Autodesk Fusion 360 part; units mm, degrees
(part 2 of 2)
sketch "Sketch1 (2)" plane through (5.45, -12.4, 0) normal (0, 1, 0) x (-1, 0, 0) in component "ServoTrayMount"
  line L0 (-16.2, -6.2) -> (-11.2, -6.2) construction
  line L1 (-16.2, 6.2) -> (-16.2, -6.2) construction
  line L2 (-16.2, -0.6) -> (-15.053256, -0.6) construction
  line L3 (-16.2, 0.6) -> (-15.053256, 0.6) construction
  circle A0 centre (-13.9, 0) radius 1.3
  line L4 (-11.2, 6.2) -> (-16.2, 6.2) construction
  line L5 (-11.2, 0) -> (-11.2, 12.4) construction
  line L6 (-11.2, 0) -> (-11.2, -12.4) construction
  line L7 (11.2, -6.2) -> (11.2, 0) construction
  line L8 (16.2, -6.2) -> (11.2, -6.2) construction
  line L9 (16.2, 6.2) -> (16.2, -6.2) construction
  line L10 (16.2, 0.6) -> (15.053256, 0.6) construction
  line L11 (16.2, -0.6) -> (15.053256, -0.6) construction
  circle A1 centre (13.9, 0) radius 1.3
  line L12 (11.2, 6.2) -> (11.2, 0) construction
  line L13 (11.2, 6.2) -> (16.2, 6.2) construction
  line L14 (-11.2, 6.2) -> (11.2, 6.2) construction
  line L15 (-11.2, -6.2) -> (11.2, -6.2) construction
  circle A2 centre (5.45, 0) radius 1.25
  line L16 (-16.2, -6.2) -> (-16.2, -6.4) construction
  line L17 (-16.2, -6.4) -> (-16.4, -6.4) construction
  line L18 (16.2, 6.2) -> (16.2, 6.4) construction
  line L19 (16.2, 6.4) -> (16.4, 6.4) construction
  line L20 (16.4, 6.4) -> (-16.4, 6.4)
  line L21 (-16.4, 6.4) -> (-16.4, -6.4)
  line L22 (-16.4, -6.4) -> (16.4, -6.4)
  line L23 (16.4, -6.4) -> (16.4, 6.4)
  line L24 (-16.4, -6.4) -> (-16.4, -9.4) construction
  line L25 (-11.2, -6.4) -> (-11.4, -6.4)
  line L26 (-11.4, -6.4) -> (-11.4, 6.4)
  line L27 (0, -6.2) -> (0, 6.2) construction
  line L28 (11.4, -6.4) -> (11.4, 6.4)
  line L29 (-16.4, -9.4) -> (-15.4, -9.4)
  line L30 (-15.4, -9.4) -> (-16.2, -9.4)
  line L31 (15.4, -9.4) -> (16.2, -9.4)
  line L32 (-16.2, 0) -> (16.2, 0) construction
  line L33 (15.4, 9.4) -> (16.2, 9.4)
  line L34 (16.2, 9.4) -> (-16.2, 9.4)
  line L35 (-16.2, 9.4) -> (-16.2, -9.4)
  line L36 (-16.2, -9.4) -> (16.2, -9.4)
  line L37 (16.2, -9.4) -> (16.2, 9.4)
  dimension "TrayGap" = 0.2
  dimension "d123" = 0.2
  dimension "d124" = 0.2
  dimension "d125" = 0.2
  dimension "TraySideWidth" = 3
  dimension "d127" = 0.2
  dimension "d128" = 1
  dimension "TrayEndExtraMinus1" = 0.8
  constraint coincident L0.start L1.end
  constraint vertical L16
  constraint perpendicular L16 L17
  constraint coincident L9.start L13.end
  constraint perpendicular L13 L18
  constraint perpendicular L18 L19
  constraint horizontal L20
  constraint vertical L21
  constraint horizontal L22
  constraint vertical L23
  constraint perpendicular L17 L24
  constraint coincident L6 L25.start
  constraint coincident L22 L25.start
  constraint perpendicular L6 L25
  constraint coincident L20 L26.end
  constraint perpendicular L20 L26
  constraint midpoint L15 L27.start
  constraint midpoint L14 L27.end
  constraint symmetric L25.end L27 L28.start
  constraint symmetric L26.end L27 L28.end
  constraint perpendicular L24 L29
  constraint parallel L29 L30
  constraint symmetric L27 L29.end L31.start
  constraint symmetric L27 L30.end L31.end
  constraint midpoint L1 L32.start
  constraint midpoint L9 L32.end
  constraint symmetric L31.start L32 L33.start
  constraint symmetric L31.end L32 L33.end
  constraint horizontal L34
  constraint vertical L35
  constraint horizontal L36
  constraint vertical L37
  measures "TrayGap" distance of L0.start L16.end
  measures "d123" distance of L16.end L17.end
  measures "d124" distance of L9.start L18.end
  measures "d125" distance of L18.end L19.end
  measures "TraySideWidth" distance of L17.end L24.end
  measures "d127" distance of L25.start L25.end
  measures "d128" distance of L24.end L29.end
  measures "TrayEndExtraMinus1" distance of L29.end L30.end
extrude "Extrude1''" add sketch "Sketch1 (2)" along normal blind 3 separate body contours L20 L33 L34 L35 L37 | L20 L22 L28 L37 | L20 L22 L26 L35 | L22 L25 L29 L30 L31 L35 L36 L37 picked at (-4.066667, 8.4) picked at (13.80095, -4.698788) picked at (-13.80095, 4.698788) picked at (-3.733333, -8.4) makes body 10 in component "ServoTrayMount"
sketch "Sketch2" plane through (0, 0, 0) normal (0, 1, 0) x (-1, 0, 0) in component "Horn"
  circle A0 centre (0, 0) radius 3.65
  circle A1 centre (8.775, 0) radius 1
  line L0 (0, 0) -> (18.1, 0)
  line L1 (0, 0) -> (0, -9.5)
  circle A2 centre (11.25, 0) radius 1
  spline S0 degree 5 poles (0, -3.65) (0.437785, -3.65) (1.360743, -3.629192) (2.887166, -3.535592) (5.121486, -3.28527) (7.811769, -2.706023) (9.437884, -1.925008) (10.102265, -1.079226) (10.25, -0.381992) (10.25, 0) knots 0 0 0 0 0 0 0.2 0.4 0.6 0.8 1 1 1 1 1 1
  line L2 (-1.091769, -3.65) -> (1.091769, -3.65)
  line L3 (10.25, -0.735761) -> (10.25, 0.735761)
  spline S1 degree 5 poles (0, 3.65) (0.437785, 3.65) (1.360743, 3.629192) (2.887166, 3.535592) (5.121486, 3.28527) (7.811769, 2.706023) (9.437884, 1.925008) (10.102265, 1.079226) (10.25, 0.381992) (10.25, 0) knots 0 0 0 0 0 0 0.2 0.4 0.6 0.8 1 1 1 1 1 1
  line L4 (-1.091769, 3.65) -> (1.091769, 3.65)
  line L5 (10.25, 0.735761) -> (10.25, -0.735761)
  line L6 (0, 0) -> (0, 9.5)
  constraint coincident L1 S0.start
  constraint coincident A0 S0.start
  constraint coincident A2 S0.end
  constraint coincident L0 S0.end
  constraint midpoint S0.start L2
  constraint horizontal L2
  constraint midpoint S0.end L3
  constraint vertical L3
  constraint symmetric L0 A0.centre L1.start
  constraint symmetric L0 L1.end L6.end
  constraint symmetric L0 S0.start S1.start
  constraint symmetric L0 S0.end S1.end
extrude "Extrude5''" add sketch "Sketch2" along normal blind 4.7 separate body contours A0 A1 L0 S0 | A0 A1 L0 S1 picked at (5.95045, -1.256119) picked at (5.95045, 1.256119) makes body 11 in component "Horn"
extrude "Extrude6" add sketch "Horn" along normal blind 4.7 contours S0 S1 S2 S3 S4 S5 S6 S7 S14 S15 S16 S17 S18 S19 S20 S21 S22 S23 S24 S25 S26 S27 S34 S35 S36 S37 S38 S39 L14 L27 | S0 S1 S2 S3 S4 S5 S6 S7 S34 S35 S36 S37 S38 S39 A5 L14 L27 | S27 S28 S29 S30 S31 S32 S33 S34 A5 L27 | S27 S28 S29 S30 S31 S32 S33 S34 L27 | S14 S15 S16 S17 S18 S19 S20 S21 S22 S23 S24 S25 S26 S27 A5 L14 L27 | S7 S8 S9 S10 S11 S12 S13 S14 L14 | S7 S8 S9 S10 S11 S12 S13 S14 A5 L14 picked at (-1.75, 0) picked at (-1.24671, 2.493427) picked at (2.756946, 0.413014) picked at (2.077276, 0.117326) picked at (1.24671, -2.493427) picked at (-2.077276, -0.117326) picked at (-2.756946, -0.413014) bodies 11 in component "Horn"
extrude "Extrude7" cut sketch "Horn" along normal blind 3.5 contours S0 S1 S2 S3 S4 S5 S6 S7 S14 S15 S16 S17 S18 S19 S20 S21 S22 S23 S24 S25 S26 S27 S34 S35 S36 S37 S38 S39 L14 L27 | S27 S28 S29 S30 S31 S32 S33 S34 L27 | S7 S8 S9 S10 S11 S12 S13 S14 L14 picked at (-1.75, 0) picked at (2.077276, 0.117326) picked at (-2.077276, -0.117326) bodies 11 in component "Horn"
move_body "Move1" bodies 11 to x (1, 0, 0) y (0, 0, -1) z (0, 1, 0) at (0, 9.5, -9.5) in component "Horn"
fillet "Fillet1" radius 0.2 40 edges at (-1.772034, 7.992148, -9.5) (-1.981642, 8.280648, -9.5) (-2.151256, 8.613536, -9.5) (-2.261454, 8.952688, -9.5) (-2.319899, 9.321697, -9.5) (-2.319899, 9.678303, -9.5) (-2.261454, 10.047312, -9.5) (-2.151256, 10.386464, -9.5) (-1.981642, 10.719352, -9.5) (-1.772034, 11.007852, -9.5) (-1.507852, 11.272034, -9.5) (-1.219352, 11.481642, -9.5) (-0.886464, 11.651256, -9.5) (-0.547312, 11.761454, -9.5) (-0.178303, 11.819899, -9.5) (0.178303, 11.819899, -9.5) (0.547312, 11.761454, -9.5) (0.886464, 11.651256, -9.5) (1.219352, 11.481642, -9.5) (1.507852, 11.272034, -9.5) (1.772034, 11.007852, -9.5) (1.981642, 10.719352, -9.5) (2.151256, 10.386464, -9.5) (2.261454, 10.047312, -9.5) (2.319899, 9.678303, -9.5) (2.319899, 9.321697, -9.5) (2.261454, 8.952688, -9.5) (2.151256, 8.613536, -9.5) (1.981642, 8.280648, -9.5) (1.772034, 7.992148, -9.5) (1.507852, 7.727966, -9.5) (1.219352, 7.518358, -9.5) (0.886464, 7.348744, -9.5) (0.547312, 7.238546, -9.5) (0.178303, 7.180101, -9.5) (-0.178303, 7.180101, -9.5) (-0.547312, 7.238546, -9.5) (-0.886464, 7.348744, -9.5) (-1.219352, 7.518358, -9.5) (-1.507852, 7.727966, -9.5) on bodies 11 in component "Horn"
sketch "HornSlottedHole" plane through (0, 0, 0) normal (0, 1, 0) x (-1, 0, 0) in component "Shaft"
  circle A0 centre (0, 0) radius 2.25 construction
  circle A1 centre (0, 0) radius 2.4 construction
  line L0 (0.347644, -2.194939) -> (0.375443, -2.370452) construction
  line L1 (0, 0) -> (0, -2.4) construction
  line L2 (-0.351978, -2.222299) -> (0, 0) construction
  line L3 (0, 0) -> (0.741641, -2.282536) construction
  line L4 (0.351978, -2.222299) -> (1.537204, -2.034577) construction
  line L5 (0, -2.4) -> (4, -2.4) construction
  circle A2 centre (0, 0) radius 2.425 construction
  circle A3 centre (0, 0) radius 2.575 construction
  line L6 (0, 0) -> (0, -2.575) construction
  line L7 (0.741641, -2.282536) -> (0.795719, -2.448971) construction
  line L8 (0.375443, -2.370452) -> (0.402819, -2.543297) construction
  spline S0 degree 5 poles (0, -2.575) (0.019371, -2.575) (0.056075, -2.571742) (0.105027, -2.557092) (0.160439, -2.521678) (0.223503, -2.466544) (0.277875, -2.427033) (0.325352, -2.406574) (0.360731, -2.398094) (0.379354, -2.395144) knots 0 0 0 0 0 0 0.2 0.4 0.6 0.8 1 1 1 1 1 1
  line L9 (-0.047124, -2.575) -> (0.047124, -2.575)
  line L10 (0.33281, -2.402516) -> (0.425897, -2.387772)
  spline S1 degree 5 poles (0, -2.575) (-0.019371, -2.575) (-0.056075, -2.571742) (-0.105027, -2.557092) (-0.160439, -2.521678) (-0.223503, -2.466544) (-0.277875, -2.427033) (-0.325352, -2.406574) (-0.360731, -2.398094) (-0.379354, -2.395144) knots 0 0 0 0 0 0 0.2 0.4 0.6 0.8 1 1 1 1 1 1
  line L11 (0.047124, -2.575) -> (-0.047124, -2.575)
  line L12 (-0.33281, -2.402516) -> (-0.425897, -2.387772)
  spline S2 degree 5 poles (0.795719, -2.448971) (0.814141, -2.442985) (0.848043, -2.428544) (0.890071, -2.399484) (0.931828, -2.34868) (0.974768, -2.276757) (1.014269, -2.222377) (1.053101, -2.188249) (1.084128, -2.169251) (1.100927, -2.160691) knots 0 0 0 0 0 0 0.2 0.4 0.6 0.8 1 1 1 1 1 1
  spline S3 degree 5 poles (0.795719, -2.448971) (0.777296, -2.454956) (0.741381, -2.4632) (0.690298, -2.464394) (0.626655, -2.447836) (0.54964, -2.414889) (0.48572, -2.394113) (0.434244, -2.389328) (0.397976, -2.392195) (0.379354, -2.395144) knots 0 0 0 0 0 0 0.2 0.4 0.6 0.8 1 1 1 1 1 1
  spline S4 degree 5 poles (1.513547, -2.083219) (1.529218, -2.071833) (1.556998, -2.047623) (1.587989, -2.006997) (1.612003, -1.945777) (1.630616, -1.864104) (1.65138, -1.80018) (1.677765, -1.755722) (1.701402, -1.728066) (1.714734, -1.714734) knots 0 0 0 0 0 0 0.2 0.4 0.6 0.8 1 1 1 1 1 1
  spline S5 degree 5 poles (1.513547, -2.083219) (1.497876, -2.094605) (1.466266, -2.113543) (1.418052, -2.130464) (1.352407, -2.134384) (1.268981, -2.126848) (1.201769, -2.126842) (1.151333, -2.138197) (1.117726, -2.152131) (1.100927, -2.160691) knots 0 0 0 0 0 0 0.2 0.4 0.6 0.8 1 1 1 1 1 1
  spline S6 degree 5 poles (2.083219, -1.513547) (2.094605, -1.497876) (2.113543, -1.466266) (2.130464, -1.418052) (2.134384, -1.352407) (2.126848, -1.268981) (2.126842, -1.201769) (2.138197, -1.151333) (2.152131, -1.117726) (2.160691, -1.100927) knots 0 0 0 0 0 0 0.2 0.4 0.6 0.8 1 1 1 1 1 1
  spline S7 degree 5 poles (2.083219, -1.513547) (2.071833, -1.529218) (2.047623, -1.556998) (2.006997, -1.587989) (1.945777, -1.612003) (1.864104, -1.630616) (1.80018, -1.65138) (1.755722, -1.677765) (1.728066, -1.701402) (1.714734, -1.714734) knots 0 0 0 0 0 0 0.2 0.4 0.6 0.8 1 1 1 1 1 1
  spline S8 degree 5 poles (2.448971, -0.795719) (2.454956, -0.777296) (2.4632, -0.741381) (2.464394, -0.690298) (2.447836, -0.626655) (2.414889, -0.54964) (2.394113, -0.48572) (2.389328, -0.434244) (2.392195, -0.397976) (2.395144, -0.379354) knots 0 0 0 0 0 0 0.2 0.4 0.6 0.8 1 1 1 1 1 1
  spline S9 degree 5 poles (2.448971, -0.795719) (2.442985, -0.814141) (2.428544, -0.848043) (2.399484, -0.890071) (2.34868, -0.931828) (2.276757, -0.974768) (2.222377, -1.014269) (2.188249, -1.053101) (2.169251, -1.084128) (2.160691, -1.100927) knots 0 0 0 0 0 0 0.2 0.4 0.6 0.8 1 1 1 1 1 1
  spline S10 degree 5 poles (2.575, 0) (2.575, 0.019371) (2.571742, 0.056075) (2.557092, 0.105027) (2.521678, 0.160439) (2.466544, 0.223503) (2.427033, 0.277875) (2.406574, 0.325352) (2.398094, 0.360731) (2.395144, 0.379354) knots 0 0 0 0 0 0 0.2 0.4 0.6 0.8 1 1 1 1 1 1
  spline S11 degree 5 poles (2.575, 0) (2.575, -0.019371) (2.571742, -0.056075) (2.557092, -0.105027) (2.521678, -0.160439) (2.466544, -0.223503) (2.427033, -0.277875) (2.406574, -0.325352) (2.398094, -0.360731) (2.395144, -0.379354) knots 0 0 0 0 0 0 0.2 0.4 0.6 0.8 1 1 1 1 1 1
  spline S12 degree 5 poles (2.448971, 0.795719) (2.442985, 0.814141) (2.428544, 0.848043) (2.399484, 0.890071) (2.34868, 0.931828) (2.276757, 0.974768) (2.222377, 1.014269) (2.188249, 1.053101) (2.169251, 1.084128) (2.160691, 1.100927) knots 0 0 0 0 0 0 0.2 0.4 0.6 0.8 1 1 1 1 1 1
  spline S13 degree 5 poles (2.448971, 0.795719) (2.454956, 0.777296) (2.4632, 0.741381) (2.464394, 0.690298) (2.447836, 0.626655) (2.414889, 0.54964) (2.394113, 0.48572) (2.389328, 0.434244) (2.392195, 0.397976) (2.395144, 0.379354) knots 0 0 0 0 0 0 0.2 0.4 0.6 0.8 1 1 1 1 1 1
  spline S14 degree 5 poles (2.083219, 1.513547) (2.071833, 1.529218) (2.047623, 1.556998) (2.006997, 1.587989) (1.945777, 1.612003) (1.864104, 1.630616) (1.80018, 1.65138) (1.755722, 1.677765) (1.728066, 1.701402) (1.714734, 1.714734) knots 0 0 0 0 0 0 0.2 0.4 0.6 0.8 1 1 1 1 1 1
  spline S15 degree 5 poles (2.083219, 1.513547) (2.094605, 1.497876) (2.113543, 1.466266) (2.130464, 1.418052) (2.134384, 1.352407) (2.126848, 1.268981) (2.126842, 1.201769) (2.138197, 1.151333) (2.152131, 1.117726) (2.160691, 1.100927) knots 0 0 0 0 0 0 0.2 0.4 0.6 0.8 1 1 1 1 1 1
  spline S16 degree 5 poles (1.513547, 2.083219) (1.497876, 2.094605) (1.466266, 2.113543) (1.418052, 2.130464) (1.352407, 2.134384) (1.268981, 2.126848) (1.201769, 2.126842) (1.151333, 2.138197) (1.117726, 2.152131) (1.100927, 2.160691) knots 0 0 0 0 0 0 0.2 0.4 0.6 0.8 1 1 1 1 1 1
  spline S17 degree 5 poles (1.513547, 2.083219) (1.529218, 2.071833) (1.556998, 2.047623) (1.587989, 2.006997) (1.612003, 1.945777) (1.630616, 1.864104) (1.65138, 1.80018) (1.677765, 1.755722) (1.701402, 1.728066) (1.714734, 1.714734) knots 0 0 0 0 0 0 0.2 0.4 0.6 0.8 1 1 1 1 1 1
  spline S18 degree 5 poles (0.795719, 2.448971) (0.777296, 2.454956) (0.741381, 2.4632) (0.690298, 2.464394) (0.626655, 2.447836) (0.54964, 2.414889) (0.48572, 2.394113) (0.434244, 2.389328) (0.397976, 2.392195) (0.379354, 2.395144) knots 0 0 0 0 0 0 0.2 0.4 0.6 0.8 1 1 1 1 1 1
  spline S19 degree 5 poles (0.795719, 2.448971) (0.814141, 2.442985) (0.848043, 2.428544) (0.890071, 2.399484) (0.931828, 2.34868) (0.974768, 2.276757) (1.014269, 2.222377) (1.053101, 2.188249) (1.084128, 2.169251) (1.100927, 2.160691) knots 0 0 0 0 0 0 0.2 0.4 0.6 0.8 1 1 1 1 1 1
  spline S20 degree 5 poles (0, 2.575) (-0.019371, 2.575) (-0.056075, 2.571742) (-0.105027, 2.557092) (-0.160439, 2.521678) (-0.223503, 2.466544) (-0.277875, 2.427033) (-0.325352, 2.406574) (-0.360731, 2.398094) (-0.379354, 2.395144) knots 0 0 0 0 0 0 0.2 0.4 0.6 0.8 1 1 1 1 1 1
  spline S21 degree 5 poles (0, 2.575) (0.019371, 2.575) (0.056075, 2.571742) (0.105027, 2.557092) (0.160439, 2.521678) (0.223503, 2.466544) (0.277875, 2.427033) (0.325352, 2.406574) (0.360731, 2.398094) (0.379354, 2.395144) knots 0 0 0 0 0 0 0.2 0.4 0.6 0.8 1 1 1 1 1 1
  spline S22 degree 5 poles (-0.795719, 2.448971) (-0.814141, 2.442985) (-0.848043, 2.428544) (-0.890071, 2.399484) (-0.931828, 2.34868) (-0.974768, 2.276757) (-1.014269, 2.222377) (-1.053101, 2.188249) (-1.084128, 2.169251) (-1.100927, 2.160691) knots 0 0 0 0 0 0 0.2 0.4 0.6 0.8 1 1 1 1 1 1
  spline S23 degree 5 poles (-0.795719, 2.448971) (-0.777296, 2.454956) (-0.741381, 2.4632) (-0.690298, 2.464394) (-0.626655, 2.447836) (-0.54964, 2.414889) (-0.48572, 2.394113) (-0.434244, 2.389328) (-0.397976, 2.392195) (-0.379354, 2.395144) knots 0 0 0 0 0 0 0.2 0.4 0.6 0.8 1 1 1 1 1 1
  spline S24 degree 5 poles (-1.513547, 2.083219) (-1.529218, 2.071833) (-1.556998, 2.047623) (-1.587989, 2.006997) (-1.612003, 1.945777) (-1.630616, 1.864104) (-1.65138, 1.80018) (-1.677765, 1.755722) (-1.701402, 1.728066) (-1.714734, 1.714734) knots 0 0 0 0 0 0 0.2 0.4 0.6 0.8 1 1 1 1 1 1
  spline S25 degree 5 poles (-1.513547, 2.083219) (-1.497876, 2.094605) (-1.466266, 2.113543) (-1.418052, 2.130464) (-1.352407, 2.134384) (-1.268981, 2.126848) (-1.201769, 2.126842) (-1.151333, 2.138197) (-1.117726, 2.152131) (-1.100927, 2.160691) knots 0 0 0 0 0 0 0.2 0.4 0.6 0.8 1 1 1 1 1 1
  spline S26 degree 5 poles (-2.083219, 1.513547) (-2.094605, 1.497876) (-2.113543, 1.466266) (-2.130464, 1.418052) (-2.134384, 1.352407) (-2.126848, 1.268981) (-2.126842, 1.201769) (-2.138197, 1.151333) (-2.152131, 1.117726) (-2.160691, 1.100927) knots 0 0 0 0 0 0 0.2 0.4 0.6 0.8 1 1 1 1 1 1
  spline S27 degree 5 poles (-2.083219, 1.513547) (-2.071833, 1.529218) (-2.047623, 1.556998) (-2.006997, 1.587989) (-1.945777, 1.612003) (-1.864104, 1.630616) (-1.80018, 1.65138) (-1.755722, 1.677765) (-1.728066, 1.701402) (-1.714734, 1.714734) knots 0 0 0 0 0 0 0.2 0.4 0.6 0.8 1 1 1 1 1 1
  spline S28 degree 5 poles (-2.448971, 0.795719) (-2.454956, 0.777296) (-2.4632, 0.741381) (-2.464394, 0.690298) (-2.447836, 0.626655) (-2.414889, 0.54964) (-2.394113, 0.48572) (-2.389328, 0.434244) (-2.392195, 0.397976) (-2.395144, 0.379354) knots 0 0 0 0 0 0 0.2 0.4 0.6 0.8 1 1 1 1 1 1
  spline S29 degree 5 poles (-2.448971, 0.795719) (-2.442985, 0.814141) (-2.428544, 0.848043) (-2.399484, 0.890071) (-2.34868, 0.931828) (-2.276757, 0.974768) (-2.222377, 1.014269) (-2.188249, 1.053101) (-2.169251, 1.084128) (-2.160691, 1.100927) knots 0 0 0 0 0 0 0.2 0.4 0.6 0.8 1 1 1 1 1 1
  spline S30 degree 5 poles (-2.575, 0) (-2.575, -0.019371) (-2.571742, -0.056075) (-2.557092, -0.105027) (-2.521678, -0.160439) (-2.466544, -0.223503) (-2.427033, -0.277875) (-2.406574, -0.325352) (-2.398094, -0.360731) (-2.395144, -0.379354) knots 0 0 0 0 0 0 0.2 0.4 0.6 0.8 1 1 1 1 1 1
  spline S31 degree 5 poles (-2.575, 0) (-2.575, 0.019371) (-2.571742, 0.056075) (-2.557092, 0.105027) (-2.521678, 0.160439) (-2.466544, 0.223503) (-2.427033, 0.277875) (-2.406574, 0.325352) (-2.398094, 0.360731) (-2.395144, 0.379354) knots 0 0 0 0 0 0 0.2 0.4 0.6 0.8 1 1 1 1 1 1
  spline S32 degree 5 poles (-2.448971, -0.795719) (-2.442985, -0.814141) (-2.428544, -0.848043) (-2.399484, -0.890071) (-2.34868, -0.931828) (-2.276757, -0.974768) (-2.222377, -1.014269) (-2.188249, -1.053101) (-2.169251, -1.084128) (-2.160691, -1.100927) knots 0 0 0 0 0 0 0.2 0.4 0.6 0.8 1 1 1 1 1 1
  spline S33 degree 5 poles (-2.448971, -0.795719) (-2.454956, -0.777296) (-2.4632, -0.741381) (-2.464394, -0.690298) (-2.447836, -0.626655) (-2.414889, -0.54964) (-2.394113, -0.48572) (-2.389328, -0.434244) (-2.392195, -0.397976) (-2.395144, -0.379354) knots 0 0 0 0 0 0 0.2 0.4 0.6 0.8 1 1 1 1 1 1
  spline S34 degree 5 poles (-2.083219, -1.513547) (-2.071833, -1.529218) (-2.047623, -1.556998) (-2.006997, -1.587989) (-1.945777, -1.612003) (-1.864104, -1.630616) (-1.80018, -1.65138) (-1.755722, -1.677765) (-1.728066, -1.701402) (-1.714734, -1.714734) knots 0 0 0 0 0 0 0.2 0.4 0.6 0.8 1 1 1 1 1 1
  spline S35 degree 5 poles (-2.083219, -1.513547) (-2.094605, -1.497876) (-2.113543, -1.466266) (-2.130464, -1.418052) (-2.134384, -1.352407) (-2.126848, -1.268981) (-2.126842, -1.201769) (-2.138197, -1.151333) (-2.152131, -1.117726) (-2.160691, -1.100927) knots 0 0 0 0 0 0 0.2 0.4 0.6 0.8 1 1 1 1 1 1
  spline S36 degree 5 poles (-1.513547, -2.083219) (-1.497876, -2.094605) (-1.466266, -2.113543) (-1.418052, -2.130464) (-1.352407, -2.134384) (-1.268981, -2.126848) (-1.201769, -2.126842) (-1.151333, -2.138197) (-1.117726, -2.152131) (-1.100927, -2.160691) knots 0 0 0 0 0 0 0.2 0.4 0.6 0.8 1 1 1 1 1 1
  spline S37 degree 5 poles (-1.513547, -2.083219) (-1.529218, -2.071833) (-1.556998, -2.047623) (-1.587989, -2.006997) (-1.612003, -1.945777) (-1.630616, -1.864104) (-1.65138, -1.80018) (-1.677765, -1.755722) (-1.701402, -1.728066) (-1.714734, -1.714734) knots 0 0 0 0 0 0 0.2 0.4 0.6 0.8 1 1 1 1 1 1
  spline S38 degree 5 poles (-0.795719, -2.448971) (-0.777296, -2.454956) (-0.741381, -2.4632) (-0.690298, -2.464394) (-0.626655, -2.447836) (-0.54964, -2.414889) (-0.48572, -2.394113) (-0.434244, -2.389328) (-0.397976, -2.392195) (-0.379354, -2.395144) knots 0 0 0 0 0 0 0.2 0.4 0.6 0.8 1 1 1 1 1 1
  spline S39 degree 5 poles (-0.795719, -2.448971) (-0.814141, -2.442985) (-0.848043, -2.428544) (-0.890071, -2.399484) (-0.931828, -2.34868) (-0.974768, -2.276757) (-1.014269, -2.222377) (-1.053101, -2.188249) (-1.084128, -2.169251) (-1.100927, -2.160691) knots 0 0 0 0 0 0 0.2 0.4 0.6 0.8 1 1 1 1 1 1
  circle A4 centre (0, 0) radius 3.65
  circle A5 centre (0, 0) radius 1.45
  dimension "d149" = 4.85
  dimension "d150" = 5.15
  dimension "d151" = 0.094248
  dimension "d152" = 0.094248
  dimension "d154" = 360
  dimension "d155" = 7.3
  dimension "d162" = 2.9
  constraint coincident A0.centre A1.centre
  constraint coincident A3 L6.end
  constraint perpendicular L5 L6
  constraint parallel L3 L7
  constraint parallel L0 L8
  constraint midpoint L6.end L9
  constraint parallel L5 L9
  constraint parallel L4 L10
  constraint symmetric S0.start L6 S1.start
  measures "d149" diameter of A2
  measures "d150" diameter of A3
  measures "d155" diameter of A4
  measures "d162" diameter of A5
extrude "Extrude6'" add sketch "HornSlottedHole" along normal blind 3.3 separate body contours A4 picked at (1.859585, 2.706557) makes body 12 in component "Shaft"
extrude "Extrude7'" add sketch "HornSlottedHole" along normal blind 4.5 and the other way blind -3.3 contours S0 S1 S2 S3 S4 S5 S6 S7 S8 S9 S10 S11 S12 S13 S14 S15 S16 S17 S18 S19 S20 S21 S22 S23 S24 S25 S26 S27 S28 S29 S30 S31 S32 S33 S34 S35 S36 S37 S38 S39 | A4 picked at (-2.101164, 0) picked at (1.859585, 2.706557) bodies 12 in component "Shaft"
move_body "Move2" bodies 12 to x (1, 0, 0) y (0, 1, 0) z (0, 0, 1) at (0, -3.3, 0) in component "Shaft"
sketch "스케치1" plane through (0, 0, 0) normal (0, 1, 0) x (1, 0, 0)
  line L0 (16.85, 6.4) -> (16.85, -6.4)
  line L1 (21.65, 9.4) -> (-10.75, 9.4)
  line L2 (16.85, -6.4) -> (-5.95, -6.4)
  line L3 (21.65, -9.4) -> (21.65, 9.4)
  circle A0 centre (-8.45, 0) radius 1.3
  line L4 (-5.95, -6.4) -> (-5.95, 6.4)
  circle A1 centre (16.2, 0) radius 1
  line L5 (16.65, 6.2) -> (-5.75, 6.2)
  point P0 (5.45, -6.2)
  dimension "d170" = 12.8
  dimension "d171" = 32.4
  dimension "d172" = 22.8
  dimension "d173" = 18.8
  dimension "d174" = 2.6
  dimension "d175" = 2.5
  dimension "d176" = 16.2
  dimension "d177" = 5.95
  dimension "d178" = 16.85
  dimension "d179" = 6.2
  dimension "d180" = 6.2
  measures "d170" distance of L0.start L0.end
  measures "d171" distance of L1.start L1.end
  measures "d172" distance of L0.end L2.end
  measures "d173" distance of L1.start L3.start
  measures "d174" diameter of A0
  measures "d175" distance of A0.centre L4
  measures "d176" distance of origin A1.centre
  measures "d177" distance of L4 origin
  measures "d178" distance of L0 origin
  measures "d179" distance of origin L5
  measures "d180" vertical distance of origin P0
sketch "스케치2" plane through (0, -9.4, 0) normal (0, 1, 0) x (-1, 0, 0)
  line L0 (5.95, 6.4) -> (5.95, -6.4)
  line L1 (-16.85, -6.4) -> (-16.85, 6.4)
  circle A0 centre (8.45, 0) radius 1.3
  line L2 (10.75, -9.4) -> (10.75, 9.4)
  point P0 (8.45, 0)
  dimension "d181" = 22.8
  dimension "d182" = 2.6
  dimension "d183" = 8.45
  dimension "d184" = 10.75
  measures "d181" distance of L0 L1
  measures "d182" diameter of A0
  measures "d183" distance of P0 origin
  measures "d184" distance of origin L2
component "Servo" placed x (1, 0, 0) y (0, 1, 0) z (0, 0, 1) at (0, 0, 0)
component "Shaft" placed x (1, 0, 0) y (0, 1, 0) z (0, 0, 1) at (0, 0, 0) in component "Servo"
component "Horn" placed x (1, 0, 0) y (0, 1, 0) z (0, 0, 1) at (0, 0, 0) in component "Servo"
component "Joint" placed x (1, 0, 0) y (0, 1, 0) z (0, 0, 1) at (0, 0, 0) in component "Servo"
component "ServoTrayMount" placed x (1, 0, 0) y (0, 1, 0) z (0, 0, 1) at (0, 0, 0) in component "Servo"
hidden bodies 2 4
equation "ShaftOuterDia = 4.8 mm + tol2"
equation "ShaftSplinesInnerDia = 4.5 mm + tol2"
equation "NumSplines = 20"
equation "d7 = ShaftOuterDia / 4"
equation "SplineTipPointiness = ShaftOuterDia * PI / NumSplines / 8"
equation "SplineInnerPointiness = ShaftOuterDia * PI / NumSplines / 8"
equation "ShaftHeight = 3.5 mm"
equation "d13 = ScrewholeDia + 0.5 * ( ( ShaftSplinesInnerDia - ScrewholeDia ) )"
equation "d20 = -ShaftHeight"
equation "d22 = -ShaftHeight"
equation "d24 = NumSplines"
equation "d26 = ScrewholeDia"
equation "ShaftScrewSectionsize = 0.2 mm"
equation "ShaftScrewPitch = ShaftHeight / 0.4 mm"
equation "d30 = -ShaftHeight"
equation "d31 = -ShaftHeight"
equation "d36 = HatTipDia / 2"
equation "HatHeight = 4.5 mm"
equation "Hole_to_closest_end_dist = HatDia / 2"
equation "ServoBodyHeight = 24 mm"
equation "ServoCornerWireRecess = 3 mm"
equation "ServoTabRecess = -4.4 mm"
equation "d47 = ServoBodyWidth"
equation "d48 = ServoTabSize"
equation "d49 = ServoBodyWidth"
equation "d52 = TabScrewSize / 2"
equation "d53 = ServoBodyWidth / 2"
equation "d55 = ( ServoBodyWidth - TabScrewGapSize ) / 2"
equation "TabThickness = -2.4 mm"
equation "d61 = WireHoleHeight"
equation "d62 = WireHoleWidth / 2"
equation "d63 = WireHoleWidth"
equation "d64 = WireHoleHeight"
equation "d65 = WireHoleWidth / 4"
equation "d66 = WireHoleWidth / 4 + 0.1 mm"
equation "d67 = WireHoleWidth / 4"
equation "d68 = -WireHoleWidth"
equation "WireLenght = 5 mm"
equation "OuterHubDia = 7.3 mm + 2 * tol"
equation "MajorArmLen = 36.2 mm + 2 * tol"
equation "MinroArmLen = 19 mm + 2 * tol"
equation "TipDiaMajor = 5 mm + 2 * tol"
equation "TipDiaMinor = 4 mm + 2 * tol"
equation "d14 = DriveHole"
equation "d19 = OuterHubDia + 1.5 mm + tol + 2 * tol"
equation "d90 = OuterHubDia + 2 * tol"
equation "ReinforcerWidth = 1 mm + 2 * tol"
equation "d92 = ReinforcerWidth / 2 + tol"
equation "HornCollarDepth = -2.7 mm"
equation "HornUnderside = -1 mm"
equation "HornInnerScrewTabThickness = 1.2 mm"
equation "HornUpperHeight = 2.3 mm"
equation "d103 = HornUpperHeight / 3"
equation "HornArmTopSide = -1.5 mm"
equation "d123 = TrayGap"
equation "d124 = TrayGap"
equation "d125 = TrayGap"
equation "d127 = TrayGap"
equation "TrayEndExtraMinus1 = 1 mm - TrayGap"
equation "ServoTrayThickness = 3 mm"
equation "qty2 = 1"
equation "qty3 = 1"
equation "qty5 = 1"
equation "HornCollarGap = 0.35 mm" comment "Servo-Arm hole size adjustment tolerance"
equation "d140 = ShaftHeight + HornScrewtopThickness"
equation "d142 = ShaftHeight + HornScrewtopThickness"
equation "d144 = ShaftHeight"
equation "d149 = ShaftSplinesInnerDia + HornCollarGap"
equation "d150 = ShaftOuterDia + HornCollarGap"
equation "d151 = SplineTipPointiness"
equation "d152 = SplineInnerPointiness"
equation "d153 = NumSplines"
equation "d155 = OuterHubDia"
equation "HornToServoTopGap = 0.2 mm" comment "Subtracted from ShaftHeight"
equation "HornScrewtopScrewDiaExtra = 0.4 mm" comment "Added to ScrewHole"
equation "d160 = ShaftHeight - HornToServoTopGap"
equation "d162 = HornScrewtopScrewDiaExtra + ScrewHole"
equation "d163 = ShaftHeight - HornToServoTopGap + HornScrewtopThickness"
equation "d165 = -( ShaftHeight - HornToServoTopGap )"
equation "d168 = -( ShaftHeight - HornToServoTopGap )"
named bodies: "Ignore", "Shaft", "Thread", "ServoBody", "Signal", "Positive", "Ground", "ServoHorn", "ServoTrayMount", "HornFitTest_", "ShaftHornConnector"
